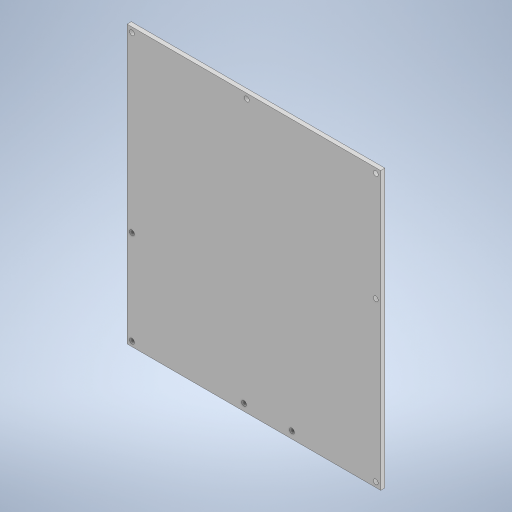
# Autodesk Inventor part: XILINX BOARD FOOTPRINT
Saved by Autodesk Inventor 2023 (Build 270158000, 158)
## iProperties
Created: 2023-04-03
Part Number: XILINX BOARD FOOTPRINT
Material: Generic
Document SubType Name: Modeling
Designer: Louis
Density: 1 g/cm^3
Appearance: Default
Author: Louis
Autodesk Inventor part; units mm, degrees
ref_plane "YZ Plane" through (0, 0, 0) normal (1, 0, 0) x (0, 1, 0)
ref_plane "XZ Plane" through (0, 0, 0) normal (0, 1, 0) x (-1, 0, 0)
ref_plane "XY Plane" through (0, 0, 0) normal (0, 0, 1) x (1, 0, 0)
sketch "Sketch1" plane through (0, 0, 0) normal (0, 0, 1) x (1, 0, 0)
  line L0 (-90, 98.25) -> (90, 98.25)
  line L1 (90, 98.25) -> (90, -98.25)
  line L2 (90, -98.25) -> (-90, -98.25)
  line L3 (-90, -98.25) -> (-90, 98.25)
  point P0 (0, 0)
  point P1 (0, 98.25)
  point P2 (-90, 0)
  dimension "d9" = 180
  dimension "d15" = 196.5
  constraints: 8 end point, 2 midpoint, 2 parallel, 1 horizontal, 1 horizontal alignment, 1 perpendicular, 1 vertical alignment
  measures "d9" distance of L0.start L0.end
  measures "d15" distance of L2.end L0.start
extrude "Extrusion1" add sketch "Sketch1" along normal blind 3
sketch "Sketch2" plane through (0, 0, 3) normal (0, 0, 1) x (1, 0, 0)
  line L0 (90, 98.25) -> (-90, 98.25) projected
  line L1 (-90, 98.25) -> (-90, -98.25) projected
  line L2 (-90, -98.25) -> (90, -98.25) projected
  line L3 (90, -98.25) -> (90, 98.25) projected
  line L4 (90, 98.25) -> (-90, 98.25) projected
  line L5 (-90, 98.25) -> (-90, -98.25) projected
  line L6 (86.5, 94.75) -> (86.5, -94.75)
  line L7 (86.5, -94.75) -> (-86.5, -94.75)
  line L8 (-86.5, -94.75) -> (-86.5, 94.75)
  line L9 (-86.5, 94.75) -> (86.5, 94.75)
  line L10 (-6.99, -93.25) -> (27, -93.25)
  point P0 (0, 0)
  point P1 (-86.5, -28.25)
  point P2 (86.5, 17.75)
  point P3 (-5, 94.75)
  dimension "d21" = 3.5
  dimension "d22" = 85
  dimension "d23" = 116
  dimension "d26" = 70
  dimension "d34" = 5
  dimension "d35" = 117
  dimension "d36" = 83.01
  constraints: 10 end point, 6 coincident, 3 point on line, 1 parallel, 3 other
  measures "d21" distance between parallel lines of L3 L6
  measures "d22" distance from line of point (-5, 94.75) L1
  measures "d23" distance from line of L2 point (86.5, 17.75)
  measures "d26" distance from line of L2 point (-86.5, -28.25)
  measures "d34" distance between parallel lines of L2 L10
  measures "d35" distance from line of L1 L10.end
  measures "d36" distance from line of L1 L10.start
hole "Hole1" at (-86.5, 94.75, 3) at (86.5, 94.75, 3) at (-86.5, -94.75, 3) at (86.5, -94.75, 3) at (-86.5, -28.25, 3) at (86.5, 17.75, 3) at (-5, 94.75, 3) at (-6.99, -93.25, 3) at (27, -93.25, 3) direction (0, 0, -1) diameter 3.4 end through all clearance for "Flat Head Machine Screw" size "M3" standard "Ansi Metric M Profile"
body "Solid1"
